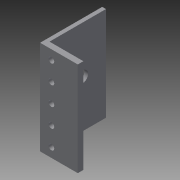
# Autodesk Inventor part: 知能ロボコンＬ字
Saved by Autodesk Inventor 2013 (Build 170138000, 138)
## iProperties
Created: 2014-05-21
Part Number: 知能ロボコンＬ字
Material: 一般
Document SubType Name: Modeling
Designer: horumo136
Density: 1 g/cm^3
Author: horumo136
Autodesk Inventor part; units mm, degrees
ref_plane "YZ Plane" through (0, 0, 0) normal (1, 0, 0) x (0, 1, 0)
ref_plane "XZ Plane" through (0, 0, 0) normal (0, 1, 0) x (-1, 0, 0)
ref_plane "XY Plane" through (0, 0, 0) normal (0, 0, 1) x (1, 0, 0)
sketch "スケッチ1" plane through (0, 0, 0) normal (0, 1, 0) x (-1, 0, 0)
  line L0 (0, 0) -> (-20, 0)
  line L1 (-20, 0) -> (-20, 50)
  line L2 (-20, 50) -> (0, 50)
  line L3 (0, 50) -> (0, 0)
  dimension "d0" = 20
  dimension "d1" = 50
  constraints: 8 end point, 2 parallel, 1 horizontal, 1 perpendicular
  measures "d0" distance of L1.end L2.end
  measures "d1" distance of L0.end L1.end
extrude "押し出し1" add sketch "スケッチ1" along normal blind 3
sketch "スケッチ2" plane through (0, 3, 0) normal (0, 1, 0) x (1, 0, 0)
  line L0 (0, -50) -> (20, -50) projected
  line L1 (0, 0) -> (2, 0)
  line L2 (2, 0) -> (2, -50)
  line L3 (2, -50) -> (0, -50)
  line L4 (0, -50) -> (0, 0)
  dimension "d4" = 2
  constraints: 8 end point, 2 parallel, 1 horizontal, 1 perpendicular, 1 point on line
  measures "d4" distance of L2.end L3.end
extrude "押し出し2" add sketch "スケッチ2" along normal blind 30
sketch "スケッチ3" plane through (2, 3, 50) normal (1, 0, 0) x (0, 0, -1)
  line L0 (50, 0) -> (0, 0) projected
  line L1 (0, 0) -> (0, 30) projected
  line L2 (25, 0) -> (25, 17.5)
  circle A0 centre (25, 17.5) radius 3
  point P0 (50, -3)
  dimension "d7" = 17.5
  dimension "d8" = 6
  constraints: 2 end point, 1 centre point, 1 coincident, 1 midpoint, 1 parallel
  measures "d7" distance of L2.start L2.end
  measures "d8" diameter of A0
hole "穴1" at (2, 20.5, 25) direction (-1, 0, 0) diameter 6 depth 8 tip angle 118
sketch "スケッチ4" plane through (0, 3, 0) normal (0, 1, 0) x (1, 0, 0)
  line L0 (20, -50) -> (20, 0) projected
  line L1 (20, 0) -> (2, 0) projected
  line L2 (20, -25) -> (6, -25)
  line L3 (6, -25) -> (6, -15)
  line L4 (6, -15) -> (6, -5)
  point P0 (0, 0)
  point P1 (6, -45)
  point P2 (6, -35)
  point P3 (6, -45)
  dimension "d16" = 14
  dimension "d17" = 10
  dimension "d18" = 10
  constraints: 6 end point, 4 coincident, 2 symmetric about line, 1 collinear, 1 midpoint, 1 parallel, 1 perpendicular
  measures "d16" distance of L2.start L2.end
  measures "d17" distance of L2.end L3.end
  measures "d18" distance of L3.end L4.end
hole "穴2" at (6, 3, 5) at (6, 3, 15) at (6, 3, 25) at (6, 3, 35) at (6, 3, 45) direction (0, -1, 0) diameter 3 depth 8 tip angle 118
